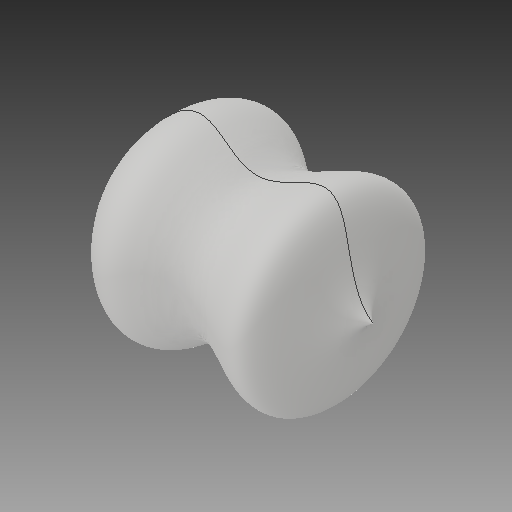
# Autodesk Inventor part: MoldPart
Saved by Autodesk Inventor 2018 (Build 220112000, 112)
## iProperties
Created: 2017-07-14
Part Number: MoldPart
Material: Типовые
Document SubType Name: Modeling
Designer: user
Density: 1 g/cm^3
Appearance: По умолчанию
Author: user
Autodesk Inventor part; units mm, degrees
ref_plane "YZ Plane" through (0, 0, 0) normal (1, 0, 0) x (0, 1, 0)
ref_plane "XZ Plane" through (0, 0, 0) normal (0, 1, 0) x (-1, 0, 0)
ref_plane "XY Plane" through (0, 0, 0) normal (0, 0, 1) x (1, 0, 0)
sketch "Эскиз1" plane through (0, 0, 0) normal (0, 0, 1) x (1, 0, 0)
  spline S0 degree 4 poles (-50, 0) (-50.1593, 1.6799) (-50.2542, 5.0563) (-49.7249, 10.1727) (-47.691, 17.0692) (-44.3987, 23.9091) (-40.0077, 30.3916) (-34.8078, 35.9699) (-29.2377, 39.8236) (-23.7367, 41.22) (-18.592, 39.8859) (-13.7615, 36.4422) (-8.8322, 32.4848) (-3.3042, 29.8136) (3.159, 29.7496) (10.4296, 32.3194) (17.9121, 36.2271) (24.8359, 39.6111) (30.5004, 40.6763) (34.5439, 38.386) (37.155, 33.0135) (38.8745, 25.6831) (40.3701, 17.8467) (42.1999, 10.734) (44.6689, 5.017) (47.1007, 1.9972) (48.9892, 0.5686) (50, 0) knots 0 0 0 0 0 0.041667 0.083333 0.125 0.166667 0.208333 0.25 0.291667 0.333333 0.375 0.416667 0.458333 0.5 0.541667 0.583333 0.625 0.666667 0.708333 0.75 0.791667 0.833333 0.875 0.916667 0.958333 1 1 1 1 1
  line L0 (-50, 0) -> (50, 0)
  point P0 (-40, 30)
  point P1 (-20, 40)
  point P2 (0, 30)
  point P3 (30, 40)
  point P4 (40, 20)
  dimension "d0" = 0
  constraints: 2 end point, 7 other
revolve "Вращение1" add sketch "Эскиз1" angle 360 about axis through (-50, 0, 0) along (1, 0, 0)
